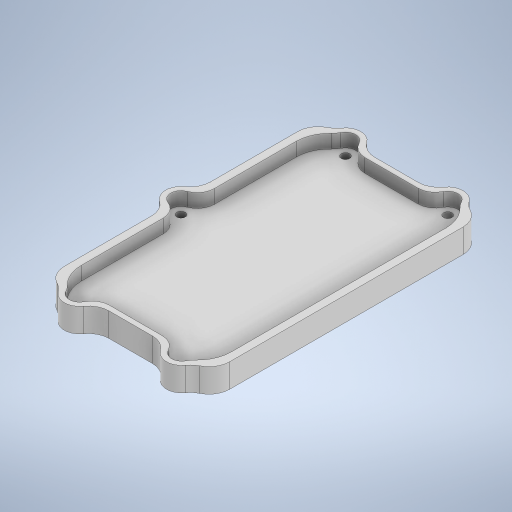
# Autodesk Inventor part: pilot_cover
Saved by Autodesk Inventor 2023 (Build 270158000, 158)
## iProperties
Created: 2023-12-11
Part Number: pilot_cover
Material: Generic
Document SubType Name: Modeling
Designer: Dawid
Density: 1 g/cm^3
Appearance: Default
Author: Dawid
Autodesk Inventor part; units mm, degrees
ref_plane "YZ Plane" through (0, 0, 0) normal (1, 0, 0) x (0, 1, 0)
ref_plane "XZ Plane" through (0, 0, 0) normal (0, 1, 0) x (-1, 0, 0)
ref_plane "XY Plane" through (0, 0, 0) normal (0, 0, 1) x (1, 0, 0)
sketch "Sketch1" plane through (0, 0, 0) normal (0, 1, 0) x (-1, 0, 0)
  circle A0 centre (0, -39) radius 1.25
  circle A1 centre (0, -39) radius 1.25
  circle A2 centre (-30, -39) radius 1.25
  circle A3 centre (-30, -39) radius 1.25
  circle A4 centre (-30, 39) radius 1.25
  circle A5 centre (-30, 39) radius 1.25
  circle A6 centre (0, 39) radius 1.25
  circle A7 centre (0, 39) radius 1.25
  arc A8 (-2.6977, -40.3125) -> (2.6984, -40.3111) centre (0, -39) ccw
  arc A9 (-32.6984, -40.3111) -> (-27.3023, -40.3125) centre (-30, -39) ccw
  circle A10 centre (9.25, 0) radius 1.25
  circle A11 centre (9.25, 0) radius 1.25
  arc A12 (10.2813, -2.8172) -> (10.2813, 2.8172) centre (9.25, 0) ccw
  arc A13 (2.6984, 40.3111) -> (-2.6977, 40.3125) centre (0, 39) ccw
  circle A14 centre (-30, 39) radius 3
  arc A15 (-27.875, -34.5) -> (-26.875, -35.5) centre (-26.875, -34.5) ccw
  arc A16 (-27.875, -34.5) -> (-26.875, -35.5) centre (-26.875, -34.5) ccw
  arc A17 (-21.875, -35.5) -> (-20.875, -34.5) centre (-21.875, -34.5) ccw
  arc A18 (-21.875, -35.5) -> (-20.875, -34.5) centre (-21.875, -34.5) ccw
  arc A19 (-9.125, -34.5) -> (-8.125, -35.5) centre (-8.125, -34.5) ccw
  arc A20 (-9.125, -34.5) -> (-8.125, -35.5) centre (-8.125, -34.5) ccw
  arc A21 (-3.125, -35.5) -> (-2.125, -34.5) centre (-3.125, -34.5) ccw
  arc A22 (-3.125, -35.5) -> (-2.125, -34.5) centre (-3.125, -34.5) ccw
  arc A23 (-8.125, 35.5) -> (-9.125, 34.5) centre (-8.125, 34.5) ccw
  arc A24 (-8.125, 35.5) -> (-9.125, 34.5) centre (-8.125, 34.5) ccw
  arc A25 (-2.125, 34.5) -> (-3.125, 35.5) centre (-3.125, 34.5) ccw
  arc A26 (-2.125, 34.5) -> (-3.125, 35.5) centre (-3.125, 34.5) ccw
  arc A27 (-20.875, 34.5) -> (-21.875, 35.5) centre (-21.875, 34.5) ccw
  arc A28 (-20.8896, 34.3297) -> (-21.875, 35.5) centre (-21.875, 34.5) ccw
  arc A29 (-26.875, 35.5) -> (-27.875, 34.5) centre (-26.875, 34.5) ccw
  arc A30 (-26.875, 35.5) -> (-27.875, 34.5) centre (-26.875, 34.5) ccw
  line L0 (-32.75, 33.5) -> (-32.75, 32.5)
  arc A31 (-32.75, 33.5) -> (-33.75, 32.5) centre (-32.75, 32.5) ccw
  line L1 (2.75, 32.5) -> (2.75, 33.5)
  arc A32 (3.75, 32.5) -> (2.75, 33.5) centre (2.75, 32.5) ccw
  line L2 (2.75, -32.5) -> (-3.625, -32.5)
  arc A33 (2.75, -33.5) -> (3.75, -32.5) centre (2.75, -32.5) ccw
  arc A34 (-33.75, -32.5) -> (-32.75, -33.5) centre (-32.75, -32.5) ccw
  arc A35 (-33.75, -32.5) -> (-32.75, -33.5) centre (-32.75, -32.5) ccw
  line L3 (-33.75, -32.5) -> (-32.75, -32.5)
  arc A36 (-32.75, 33.5) -> (-33.75, 32.5) centre (-32.75, 32.5) ccw
  line L4 (-33.75, -32.5) -> (-33.75, 32.5)
  line L5 (-32.75, 33.5) -> (-27.875, 33.5)
  line L6 (-32.75, 33.5) -> (-27.875, 33.5)
  line L7 (-27.875, 33.5) -> (-27.875, 34.5)
  line L8 (-26.875, 35.5) -> (-21.875, 35.5)
  line L9 (-22.375, 34) -> (-20.875, 34.5)
  line L10 (-20.9608, 33.5) -> (-9.0392, 33.5)
  line L11 (-20.875, 34.5) -> (-20.9608, 33.5)
  line L12 (-9.125, 33.5) -> (-9.125, 34.5)
  line L13 (-20.9608, 33.5) -> (-9.125, 33.5)
  line L14 (-9.125, 33.5) -> (-9.125, 34.5)
  line L15 (-3.125, 35.5) -> (-8.125, 35.5)
  line L16 (-8.125, 35.5) -> (-3.125, 35.5)
  line L17 (-2.125, 34.5) -> (-2.125, 33.5)
  line L18 (-2.125, 34.5) -> (-2.125, 33.5)
  line L19 (-2.125, 33.5) -> (2.75, 33.5)
  line L20 (-2.125, 33.5) -> (2.75, 33.5)
  line L21 (3.75, 32.5) -> (3.75, -32.5)
  line L22 (3.75, 32.5) -> (3.75, -32.5)
  line L23 (2.75, -33.5) -> (-2.125, -33.5)
  line L24 (-2.2108, -33.5) -> (2.75, -33.5)
  line L25 (-2.125, -34.5) -> (-2.125, -33.5)
  line L26 (-2.125, -33.5) -> (-2.125, -34.5)
  line L27 (-3.125, -35.5) -> (-8.125, -35.5)
  line L28 (-9.125, -33.5) -> (-9.125, -34.5)
  line L29 (-9.125, -34.5) -> (-9.125, -33.5)
  line L30 (-20.9608, -33.5) -> (-20.875, -33.5)
  line L31 (-9.125, -33.5) -> (-20.875, -33.5)
  line L32 (-20.875, -34.5) -> (-20.875, -33.5)
  line L33 (-20.875, -33.5) -> (-20.875, -34.5)
  line L34 (-26.875, -35.5) -> (-21.875, -35.5)
  line L35 (-26.875, -35.5) -> (-21.875, -35.5)
  line L36 (-26.375, -34) -> (-27.875, -34.5)
  line L37 (-27.875, -33.5) -> (-27.875, -34.5)
  line L38 (-27.875, -34.5) -> (-27.875, -33.5)
  line L39 (-27.7892, -33.5) -> (-32.75, -33.5)
  line L40 (-27.875, -33.5) -> (-32.75, -33.5)
  arc A37 (7, 7.5125) -> (10.2813, 2.8172) centre (12, 7.5125) ccw
  arc A38 (7, 7.5125) -> (10.2813, 2.8172) centre (12, 7.5125) ccw
  arc A39 (10.2813, -2.8172) -> (7, -7.5125) centre (12, -7.5125) ccw
  arc A40 (10.2813, -2.8172) -> (7, -7.5125) centre (12, -7.5125) ccw
  arc A41 (-2.6977, -40.3125) -> (-7.1937, -37.5) centre (-7.1937, -42.5) ccw
  arc A42 (-2.6977, -40.3125) -> (-7.1937, -37.5) centre (-7.1937, -42.5) ccw
  arc A43 (-32.6984, -40.3111) -> (-33.7971, -38.8288) centre (-37.1956, -42.4962) ccw
  arc A44 (-32.6984, -40.3111) -> (-33.7971, -38.8288) centre (-37.1956, -42.4962) ccw
  arc A45 (-22.8063, -37.5) -> (-27.3023, -40.3125) centre (-22.8063, -42.5) ccw
  arc A46 (-22.8063, -37.5) -> (-27.3023, -40.3125) centre (-22.8063, -42.5) ccw
  arc A47 (-23.7055, 42.0625) -> (-22.8063, 41.5) centre (-22.8063, 42.5) ccw
  arc A48 (-27.3023, 40.3125) -> (-22.8063, 37.5) centre (-22.8063, 42.5) ccw
  arc A49 (-7.1937, 37.5) -> (-2.6977, 40.3125) centre (-7.1937, 42.5) ccw
  line L41 (-7.1937, -37.5) -> (-22.8063, -37.5)
  line L42 (-22.8063, -37.5) -> (-7.1937, -37.5)
  line L43 (-22.8063, 37.5) -> (-7.1937, 37.5)
  line L44 (-22.8063, 37.5) -> (-7.1937, 37.5)
  arc A50 (7, 31.4939) -> (3.7971, 38.8288) centre (-3, 31.4939) ccw
  arc A51 (7, 31.4939) -> (3.7971, 38.8288) centre (-3, 31.4939) ccw
  arc A52 (2.6984, 40.3111) -> (3.7971, 38.8288) centre (7.1956, 42.4962) ccw
  arc A53 (2.6984, 40.3111) -> (3.7971, 38.8288) centre (7.1956, 42.4962) ccw
  line L45 (7, 7.5125) -> (7, 31.4939)
  line L46 (7, 31.4939) -> (7, 7.5125)
  arc A54 (3.7971, -38.8288) -> (7, -31.4939) centre (-3, -31.4939) ccw
  arc A55 (3.7971, -38.8288) -> (7, -31.4939) centre (-3, -31.4939) ccw
  arc A56 (3.2011, -39.4889) -> (2.6984, -40.3111) centre (7.1956, -42.4962) ccw
  arc A57 (3.2011, -39.4889) -> (2.6984, -40.3111) centre (7.1956, -42.4962) ccw
  arc A58 (3.7971, -38.8288) -> (2.6984, -40.3111) centre (7.1956, -42.4962) ccw
  arc A59 (3.7971, -38.8288) -> (3.2011, -39.4889) centre (7.1956, -42.4962) ccw
  line L47 (7, -31.14) -> (7, -31.4939)
  line L48 (7, -7.5125) -> (7, -31.4939)
  arc A60 (-36.2857, -35.2055) -> (-33.7971, -38.8288) centre (-27, -31.4939) ccw
  arc A61 (-36.2857, -35.2055) -> (-33.7971, -38.8288) centre (-27, -31.4939) ccw
  arc A62 (-37, -31.4939) -> (-36.2857, -35.2055) centre (-27, -31.4939) ccw
  arc A63 (-37, -31.4939) -> (-36.2857, -35.2055) centre (-27, -31.4939) ccw
  arc A64 (-33.7971, 38.8288) -> (-32.6984, 40.3111) centre (-37.1956, 42.4962) ccw
  arc A65 (-33.7971, 38.8288) -> (-37, 31.4939) centre (-27, 31.4939) ccw
  arc A66 (-33.7971, 38.8288) -> (-37, 31.4939) centre (-27, 31.4939) ccw
  arc A67 (-33.7971, 38.8288) -> (-32.6984, 40.3111) centre (-37.1956, 42.4962) ccw
  line L49 (-37, 31.4939) -> (-37, -31.4939)
  line L50 (-37, -31.4939) -> (-37, 31.4939)
  line L51 (-37, 39.3845) -> (-37, -39.3845)
  line L52 (3.75, 0) -> (-33.75, 0)
  line L53 (-33.75, 0) -> (-15, 0)
  line L54 (-44.5, 44.5) -> (14.5, 44.5)
  line L55 (14.5, 44.5) -> (14.5, -44.5)
  line L56 (14.5, -44.5) -> (-44.5, -44.5)
  line L57 (-44.5, -44.5) -> (-44.5, 44.5)
  line L58 (-44.5, 44.5) -> (14.5, -44.5) construction
  line L59 (14.5, 44.5) -> (-44.5, -44.5) construction
  point P0 (0, 0)
  dimension "d0" = 59
  dimension "d1" = 89
  constraints: 120 end point, 118 point on circle, 68 centre point, 25 coincident, 23 tangent, 14 collinear, 6 perpendicular, 5 midpoint, 3 point on line, 2 horizontal, 2 parallel, 2 vertical, 1 concentric
  measures "d0" distance of L55.end L56.end
  measures "d1" distance of L54.end L55.end
extrude "Extrusion1" add sketch "Sketch1" along normal blind 3 contours A41 L41 A45 A9 A43 A60 A62 L49 A65 A64 A14 A48 L43 A49 A13 A52 A50 L45 A37 A12 A39 L48 L47 A54 A58 A56 A8 | A14 | L37 L39 A34 L4 L52 L21 A33 L23 L25 A21 L27 A19 L28 L31 L32 A17 L34 A15 | L4 A31 L5 L7 A29 L8 A27 L11 L10 L12 A23 L15 A25 L17 L19 A32 L21 L52
sketch "Sketch2" plane through (0, 0, 0) normal (0, -1, 0) x (1, 0, 0)
  circle A0 centre (0, 39) radius 1.25
  circle A1 centre (0, 39) radius 1.25
  circle A2 centre (30, 39) radius 1.25
  circle A3 centre (30, 39) radius 1.25
  circle A4 centre (30, -39) radius 1.25
  circle A5 centre (30, -39) radius 1.25
  circle A6 centre (0, -39) radius 1.25
  circle A7 centre (0, -39) radius 1.25
  arc A8 (2.6977, 40.3125) -> (-2.6984, 40.3111) centre (0, 39) ccw
  arc A9 (32.6984, 40.3111) -> (27.3023, 40.3125) centre (30, 39) ccw
  circle A10 centre (-9.25, 0) radius 1.25
  circle A11 centre (-9.25, 0) radius 1.25
  arc A12 (-10.2813, 2.8172) -> (-10.2812, -2.8172) centre (-9.25, 0) ccw
  arc A13 (-2.6984, -40.3111) -> (2.6977, -40.3125) centre (0, -39) ccw
  arc A14 (27.3023, -40.3125) -> (32.6984, -40.3111) centre (30, -39) ccw
  arc A15 (27.875, 34.5) -> (26.875, 35.5) centre (26.875, 34.5) ccw
  arc A16 (27.875, 34.5) -> (26.875, 35.5) centre (26.875, 34.5) ccw
  arc A17 (21.875, 35.5) -> (20.875, 34.5) centre (21.875, 34.5) ccw
  arc A18 (21.875, 35.5) -> (20.875, 34.5) centre (21.875, 34.5) ccw
  arc A19 (9.125, 34.5) -> (8.125, 35.5) centre (8.125, 34.5) ccw
  arc A20 (9.125, 34.5) -> (8.125, 35.5) centre (8.125, 34.5) ccw
  arc A21 (3.125, 35.5) -> (2.125, 34.5) centre (3.125, 34.5) ccw
  arc A22 (3.125, 35.5) -> (2.125, 34.5) centre (3.125, 34.5) ccw
  arc A23 (8.125, -35.5) -> (9.125, -34.5) centre (8.125, -34.5) ccw
  arc A24 (8.125, -35.5) -> (9.125, -34.5) centre (8.125, -34.5) ccw
  arc A25 (2.125, -34.5) -> (3.125, -35.5) centre (3.125, -34.5) ccw
  arc A26 (2.125, -34.5) -> (3.125, -35.5) centre (3.125, -34.5) ccw
  arc A27 (20.875, -34.5) -> (21.875, -35.5) centre (21.875, -34.5) ccw
  arc A28 (20.8896, -34.3297) -> (21.875, -35.5) centre (21.875, -34.5) ccw
  arc A29 (26.875, -35.5) -> (27.875, -34.5) centre (26.875, -34.5) ccw
  arc A30 (26.875, -35.5) -> (27.875, -34.5) centre (26.875, -34.5) ccw
  line L0 (32.75, -33.5) -> (32.75, -32.5)
  arc A31 (32.75, -33.5) -> (33.75, -32.5) centre (32.75, -32.5) ccw
  line L1 (-2.75, -32.5) -> (-2.75, -33.5)
  arc A32 (-3.75, -32.5) -> (-2.75, -33.5) centre (-2.75, -32.5) ccw
  line L2 (-2.75, 32.5) -> (3.625, 32.5)
  arc A33 (-2.75, 33.5) -> (-3.75, 32.5) centre (-2.75, 32.5) ccw
  arc A34 (33.75, 32.5) -> (32.75, 33.5) centre (32.75, 32.5) ccw
  arc A35 (33.75, 32.5) -> (32.75, 33.5) centre (32.75, 32.5) ccw
  line L3 (33.75, 32.5) -> (32.75, 32.5)
  arc A36 (32.75, -33.5) -> (33.75, -32.5) centre (32.75, -32.5) ccw
  line L4 (33.75, 32.5) -> (33.75, -32.5)
  line L5 (32.75, -33.5) -> (27.875, -33.5)
  line L6 (32.75, -33.5) -> (27.875, -33.5)
  line L7 (27.875, -33.5) -> (27.875, -34.5)
  line L8 (26.875, -35.5) -> (21.875, -35.5)
  line L9 (22.375, -34) -> (20.875, -34.5)
  line L10 (20.9608, -33.5) -> (9.0392, -33.5)
  line L11 (20.875, -34.5) -> (20.9608, -33.5)
  line L12 (9.125, -33.5) -> (9.125, -34.5)
  line L13 (20.9608, -33.5) -> (9.125, -33.5)
  line L14 (9.125, -33.5) -> (9.125, -34.5)
  line L15 (3.125, -35.5) -> (8.125, -35.5)
  line L16 (8.125, -35.5) -> (3.125, -35.5)
  line L17 (2.125, -34.5) -> (2.125, -33.5)
  line L18 (2.125, -34.5) -> (2.125, -33.5)
  line L19 (2.125, -33.5) -> (-2.75, -33.5)
  line L20 (2.125, -33.5) -> (-2.75, -33.5)
  line L21 (-3.75, -32.5) -> (-3.75, 32.5)
  line L22 (-3.75, -32.5) -> (-3.75, 32.5)
  line L23 (-2.75, 33.5) -> (2.125, 33.5)
  line L24 (2.2108, 33.5) -> (-2.75, 33.5)
  line L25 (2.125, 34.5) -> (2.125, 33.5)
  line L26 (2.125, 33.5) -> (2.125, 34.5)
  line L27 (3.125, 35.5) -> (8.125, 35.5)
  line L28 (9.125, 33.5) -> (9.125, 34.5)
  line L29 (9.125, 34.5) -> (9.125, 33.5)
  line L30 (20.9608, 33.5) -> (20.875, 33.5)
  line L31 (9.125, 33.5) -> (20.875, 33.5)
  line L32 (20.875, 34.5) -> (20.875, 33.5)
  line L33 (20.875, 33.5) -> (20.875, 34.5)
  line L34 (26.875, 35.5) -> (21.875, 35.5)
  line L35 (26.875, 35.5) -> (21.875, 35.5)
  line L36 (26.375, 34) -> (27.875, 34.5)
  line L37 (27.875, 33.5) -> (27.875, 34.5)
  line L38 (27.875, 34.5) -> (27.875, 33.5)
  line L39 (27.7892, 33.5) -> (32.75, 33.5)
  line L40 (27.875, 33.5) -> (32.75, 33.5)
  arc A37 (-7, -7.5125) -> (-10.2812, -2.8172) centre (-12, -7.5125) ccw
  arc A38 (-7, -7.5125) -> (-10.2812, -2.8172) centre (-12, -7.5125) ccw
  arc A39 (-10.2813, 2.8172) -> (-7, 7.5125) centre (-12, 7.5125) ccw
  arc A40 (-10.2813, 2.8172) -> (-7, 7.5125) centre (-12, 7.5125) ccw
  arc A41 (2.6977, 40.3125) -> (7.1937, 37.5) centre (7.1937, 42.5) ccw
  arc A42 (2.6977, 40.3125) -> (7.1937, 37.5) centre (7.1937, 42.5) ccw
  arc A43 (32.6984, 40.3111) -> (33.7971, 38.8288) centre (37.1956, 42.4962) ccw
  arc A44 (32.6984, 40.3111) -> (33.7971, 38.8288) centre (37.1956, 42.4962) ccw
  arc A45 (22.8063, 37.5) -> (27.3023, 40.3125) centre (22.8063, 42.5) ccw
  arc A46 (22.8063, 37.5) -> (27.3023, 40.3125) centre (22.8063, 42.5) ccw
  arc A47 (23.7055, -42.0625) -> (22.8063, -41.5) centre (22.8063, -42.5) ccw
  arc A48 (27.3023, -40.3125) -> (22.8063, -37.5) centre (22.8063, -42.5) ccw
  arc A49 (7.1937, -37.5) -> (2.6977, -40.3125) centre (7.1937, -42.5) ccw
  line L41 (7.1937, 37.5) -> (22.8063, 37.5)
  line L42 (22.8063, 37.5) -> (7.1937, 37.5)
  line L43 (22.8063, -37.5) -> (7.1937, -37.5)
  line L44 (22.8063, -37.5) -> (7.1937, -37.5)
  arc A50 (-7, -31.4939) -> (-3.7971, -38.8288) centre (3, -31.4939) ccw
  arc A51 (-7, -31.4939) -> (-3.7971, -38.8288) centre (3, -31.4939) ccw
  arc A52 (-2.6984, -40.3111) -> (-3.7971, -38.8288) centre (-7.1956, -42.4962) ccw
  arc A53 (-2.6984, -40.3111) -> (-3.7971, -38.8288) centre (-7.1956, -42.4962) ccw
  line L45 (-7, -7.5125) -> (-7, -31.4939)
  line L46 (-7, -31.4939) -> (-7, -7.5125)
  arc A54 (-3.7971, 38.8288) -> (-7, 31.4939) centre (3, 31.4939) ccw
  arc A55 (-3.7971, 38.8288) -> (-7, 31.4939) centre (3, 31.4939) ccw
  arc A56 (-3.2011, 39.4889) -> (-2.6984, 40.3111) centre (-7.1956, 42.4962) ccw
  arc A57 (-3.2011, 39.4889) -> (-2.6984, 40.3111) centre (-7.1956, 42.4962) ccw
  arc A58 (-3.7971, 38.8288) -> (-2.6984, 40.3111) centre (-7.1956, 42.4962) ccw
  arc A59 (-3.7971, 38.8288) -> (-3.2011, 39.4889) centre (-7.1956, 42.4962) ccw
  line L47 (-7, 31.14) -> (-7, 31.4939)
  line L48 (-7, 7.5125) -> (-7, 31.4939)
  arc A60 (36.2857, 35.2055) -> (33.7971, 38.8288) centre (27, 31.4939) ccw
  arc A61 (36.2857, 35.2055) -> (33.7971, 38.8288) centre (27, 31.4939) ccw
  arc A62 (37, 31.4939) -> (36.2857, 35.2055) centre (27, 31.4939) ccw
  arc A63 (37, 31.4939) -> (36.2857, 35.2055) centre (27, 31.4939) ccw
  arc A64 (33.7971, -38.8288) -> (32.6984, -40.3111) centre (37.1956, -42.4962) ccw
  arc A65 (33.7971, -38.8288) -> (37, -31.4939) centre (27, -31.4939) ccw
  arc A66 (33.7971, -38.8288) -> (37, -31.4939) centre (27, -31.4939) ccw
  arc A67 (33.7971, -38.8288) -> (32.6984, -40.3111) centre (37.1956, -42.4962) ccw
  line L49 (37, -31.4939) -> (37, 31.4939)
  line L50 (37, 31.4939) -> (37, -31.4939)
  arc A68 (-8.122, -4.3563) -> (-9.25, -4.5) centre (-9.25, 0) ccw
  circle A69 centre (0, 39) radius 1.25 projected
  circle A70 centre (30, 39) radius 1.25 projected
  circle A71 centre (30, -39) radius 1.25 projected
  arc A72 (-2.6984, -40.3111) -> (2.6977, -40.3125) centre (0, -39) ccw projected
  line L51 (39.25, 39) -> (39.25, -39)
  line L52 (39.25, -39) -> (-9.25, 39) construction
  line L53 (-9.25, -39) -> (39.25, 39) construction
  line L54 (-4.5, -39) -> (-9.25, -39)
  line L55 (-9.25, -39) -> (-9.25, -4.5)
  line L56 (-9.25, -3.3367) -> (-9.25, 3.3367)
  line L57 (-9.25, 4.5) -> (-9.25, 39)
  line L58 (-9.25, 39) -> (-4.5, 39)
  line L59 (-3.6211, 39) -> (3.623, 39)
  arc A73 (-4.4266, 38.1906) -> (4.4485, 38.3211) centre (0, 39) ccw
  arc A74 (4.5, 39) -> (-4.5, 39) centre (0, 39) ccw
  arc A75 (-4.5, -39) -> (4.5, -39) centre (0, -39) ccw
  arc A76 (4.4485, -38.3211) -> (-4.4266, -38.1906) centre (0, -39) ccw
  line L60 (3.623, -39) -> (-1.25, -39)
  line L61 (25.5, -39) -> (4.5, -39)
  line L62 (39.25, -39) -> (34.5, -39)
  line L63 (33.6211, -39) -> (26.377, -39)
  arc A77 (25.5, -39) -> (34.5, -39) centre (30, -39) ccw
  arc A78 (34.4266, -38.1906) -> (25.5515, -38.3211) centre (30, -39) ccw
  line L64 (34.5, 39) -> (39.25, 39)
  line L65 (4.5, 39) -> (25.5, 39)
  line L66 (26.377, 39) -> (33.6211, 39)
  arc A79 (34.5, 39) -> (25.5, 39) centre (30, 39) ccw
  arc A80 (25.5515, 38.3211) -> (34.4266, 38.1906) centre (30, 39) ccw
  point P0 (-30, -39)
  point P1 (0, 0)
  point P2 (15, 0)
  dimension "d4" = 9
  dimension "d9" = 48.5
  constraints: 156 point on circle, 134 end point, 76 centre point, 30 coincident, 28 parallel, 23 tangent, 20 perpendicular, 13 collinear, 5 horizontal, 3 point on line, 2 midpoint, 1 concentric, 1 horizontal alignment, 2 other
  measures "d4" diameter of A68
  measures "d9" distance of L52.end L51.start
extrude "Extrusion2" add sketch "Sketch2" against normal blind 7 contours L57 L58 A74 L65 A79 L64 L51 L62 A77 L61 A75 L54 L55 A68
fillet "Fillet1" radius 6 10 edges at (-4.5, 3.5, 39) (4.5, 3.5, 39) (25.5, 3.5, 39) (34.5, 3.5, 39) (34.5, 3.5, -39) (25.5, 3.5, -39) (4.5, 3.5, -39) (-4.5, 3.5, -39) (-9.25, 3.5, -4.5) (-9.25, 3.5, 4.5)
fillet "Fillet2" radius 6 4 edges at (-9.25, 3.5, 39) (-9.25, 3.5, -39) (39.25, 3.5, -39) (39.25, 3.5, 39)
body "Solid1"
